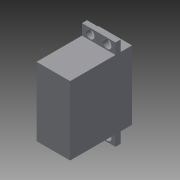
# Autodesk Inventor part: servo
Saved by Autodesk Inventor 2014 SP1 (Build 180222100, 222)
## iProperties
Created: 2014-03-28
Part Number: servo
Material: Générique
Document SubType Name: Modeling
Designer: astralien3000
Density: 1 g/cm^3
Appearance: Par défaut
length: 40,600 mm
width: 19,800 mm
axe_dist: 10,000 mm
d3: 9,900 mm
height: 36,600 mm
d5: 0,00 deg
handle_height: 26,800 mm
handle_thickness: 3,000 mm
handle_length: 6,400 mm
d9: 0,00 deg
d10: 26,800 mm
d11: 3,000 mm
d12: 6,400 mm
d13: 0,00 deg
d14: 9,900 mm
hole_dist: 5,000 mm
d16: 3,200 mm
hole_diameter: 5,000 mm
d19: 0,00 deg
d20: 9,900 mm
d21: 3,200 mm
d22: 5,000 mm
d23: 5,000 mm
d25: 0,00 deg
d26: 9,900 mm
d27: 5,000 mm
d28: 3,200 mm
d29: 5,000 mm
d31: 0,00 deg
d32: 9,900 mm
d33: 5,000 mm
d34: 5,000 mm
d35: 3,200 mm
d37: 0,00 deg
axe_diameter: 6,000 mm
axe_height: 6,700 mm
d40: 0,00 deg
d41: 10,000 mm
Author: astralien3000
Autodesk Inventor part; units mm, degrees
ref_plane "YZ Plane" through (0, 0, 0) normal (1, 0, 0) x (0, 1, 0)
ref_plane "XZ Plane" through (0, 0, 0) normal (0, 1, 0) x (-1, 0, 0)
ref_plane "XY Plane" through (0, 0, 0) normal (0, 0, 1) x (1, 0, 0)
sketch "servo_base" plane through (0, 0, 0) normal (0, 1, 0) x (-1, 0, 0)
  line L0 (-9.9, 10) -> (9.9, 10)
  line L1 (9.9, 10) -> (9.9, -30.6)
  line L2 (9.9, -30.6) -> (-9.9, -30.6)
  line L3 (-9.9, -30.6) -> (-9.9, 10)
  point P0 (0, 0)
  dimension "length" = 40.6
  dimension "width" = 19.8
  dimension "axe_dist" = 10
  dimension "d3" = 9.9
  constraints: 8 end point, 2 parallel, 1 horizontal, 1 perpendicular
  measures "length" distance of L0.end L1.end
  measures "width" distance of L0.start L0.end
  measures "axe_dist" distance from line of L0 point (0, 0)
  measures "d3" distance from line of L1 point (0, 0)
extrude "servo_body" add sketch "servo_base" along normal blind 36.6
sketch "handle1_base" plane through (-9.9, 0, 10) normal (0, 0, 1) x (1, 0, 0)
  line L0 (19.8, 0) -> (0, 0) projected
  line L1 (19.8, 0) -> (19.8, 36.6) projected
  line L2 (0, 0) -> (0, 36.6) projected
  line L3 (0, 26.8) -> (19.8, 26.8)
  line L4 (19.8, 26.8) -> (19.8, 29.8)
  line L5 (19.8, 29.8) -> (0, 29.8)
  line L6 (0, 29.8) -> (0, 26.8)
  point P0 (9.9, 0)
  dimension "handle_height" = 26.8
  dimension "handle_thickness" = 3
  constraints: 8 end point, 2 parallel, 2 point on line, 1 horizontal, 1 perpendicular
  measures "handle_height" distance between parallel lines of L0 L3
  measures "handle_thickness" distance between parallel lines of L3 L5
extrude "handle1" add sketch "handle1_base" along normal blind 6.4 contours L3 L2 L5 L1
sketch "handle2_base" plane through (9.9, 0, -30.6) normal (0, 0, -1) x (-1, 0, 0)
  line L0 (19.8, 0) -> (0, 0) projected
  line L1 (19.8, 0) -> (19.8, 36.6) projected
  line L2 (0, 0) -> (0, 36.6) projected
  line L3 (0, 26.8) -> (19.8, 26.8)
  line L4 (19.8, 26.8) -> (19.8, 29.8)
  line L5 (19.8, 29.8) -> (0, 29.8)
  line L6 (0, 29.8) -> (0, 26.8)
  point P0 (9.9, 0)
  dimension "d10" = 26.8
  dimension "d11" = 3
  constraints: 8 end point, 2 parallel, 2 point on line, 1 horizontal, 1 perpendicular
  measures "d10" distance between parallel lines of L0 L3
  measures "d11" distance between parallel lines of L3 L5
extrude "handle2" add sketch "handle2_base" along normal blind 6.4 contours L3 L2 L5 L1
sketch "hole1_right_base" plane through (-9.9, 29.8, 10) normal (0, 1, 0) x (1, 0, 0)
  line L0 (19.8, -6.4) -> (0, -6.4) projected
  line L1 (19.8, 0) -> (19.8, -6.4) projected
  line L2 (0, 0) -> (9.9, 0)
  line L3 (9.9, 0) -> (9.9, -6.4)
  line L4 (9.9, -6.4) -> (0, -6.4)
  line L5 (0, -6.4) -> (0, 0)
  circle A0 centre (4.9, -3.2) radius 2.5
  point P0 (9.9, 10)
  dimension "d14" = 9.9
  dimension "hole_dist" = 5
  dimension "d16" = 3.2
  dimension "hole_diameter" = 5
  constraints: 8 end point, 2 parallel, 1 centre point, 1 horizontal, 1 midpoint, 1 perpendicular
  measures "d14" distance between parallel lines of L1 L3
  measures "hole_dist" distance from line of L3 A0.centre
  measures "d16" distance from line of L0 A0.centre
  measures "hole_diameter" diameter of A0
extrude "hole1_rigth" cut sketch "hole1_right_base" against normal up to next contours A0
sketch "hole1_left_base" plane through (-9.9, 29.8, 10) normal (0, 1, 0) x (1, 0, 0)
  line L0 (0, 0) -> (0, -6.4) projected
  line L1 (19.8, -6.4) -> (0, -6.4) projected
  line L2 (19.8, 0) -> (9.9, 0)
  line L3 (9.9, 0) -> (9.9, -6.4)
  line L4 (9.9, -6.4) -> (19.8, -6.4)
  line L5 (19.8, -6.4) -> (19.8, 0)
  circle A0 centre (14.9, -3.2) radius 2.5
  point P0 (9.9, 10)
  dimension "d20" = 9.9
  dimension "d21" = 3.2
  dimension "d22" = 5
  dimension "d23" = 5
  constraints: 8 end point, 2 parallel, 1 centre point, 1 horizontal, 1 midpoint, 1 perpendicular
  measures "d20" distance between parallel lines of L0 L3
  measures "d21" distance from line of L1 A0.centre
  measures "d22" distance from line of L3 A0.centre
  measures "d23" diameter of A0
extrude "hole1_left" cut sketch "hole1_left_base" against normal up to next contours A0
sketch "hole2_right_base" plane through (-9.9, 29.8, -30.6) normal (0, 1, 0) x (1, 0, 0)
  line L0 (19.8, 0) -> (0, 0) projected
  line L1 (19.8, 0) -> (19.8, 6.4) projected
  line L2 (0, 6.4) -> (19.8, 6.4) projected
  line L3 (0, 6.4) -> (9.9, 6.4)
  line L4 (9.9, 6.4) -> (9.9, 0)
  line L5 (9.9, 0) -> (0, 0)
  line L6 (0, 0) -> (0, 6.4)
  circle A0 centre (4.9, 3.2) radius 2.5
  point P0 (9.9, -30.6)
  dimension "d26" = 9.9
  dimension "d27" = 5
  dimension "d28" = 3.2
  dimension "d29" = 5
  constraints: 8 end point, 2 parallel, 1 centre point, 1 horizontal, 1 midpoint, 1 perpendicular
  measures "d26" distance between parallel lines of L1 L4
  measures "d27" distance from line of L4 A0.centre
  measures "d28" distance from line of L2 A0.centre
  measures "d29" diameter of A0
extrude "hole2_right" cut sketch "hole2_right_base" against normal up to next contours A0
sketch "hole2_left_base" plane through (-9.9, 29.8, -30.6) normal (0, 1, 0) x (1, 0, 0)
  line L0 (19.8, 0) -> (0, 0) projected
  line L1 (0, 6.4) -> (19.8, 6.4) projected
  line L2 (0, 0) -> (0, 6.4) projected
  line L3 (19.8, 6.4) -> (9.9, 6.4)
  line L4 (9.9, 6.4) -> (9.9, 0)
  line L5 (9.9, 0) -> (19.8, 0)
  line L6 (19.8, 0) -> (19.8, 6.4)
  circle A0 centre (14.9, 3.2) radius 2.5
  point P0 (9.9, -30.6)
  dimension "d32" = 9.9
  dimension "d33" = 5
  dimension "d34" = 5
  dimension "d35" = 3.2
  constraints: 8 end point, 2 parallel, 1 centre point, 1 horizontal, 1 midpoint, 1 perpendicular
  measures "d32" distance between parallel lines of L2 L4
  measures "d33" diameter of A0
  measures "d34" distance from line of L4 A0.centre
  measures "d35" distance from line of L1 A0.centre
extrude "hole2_left" cut sketch "hole2_left_base" against normal up to next contours A0
sketch "axe_base" plane through (0, 36.6, 0) normal (0, 1, 0) x (1, 0, 0)
  circle A0 centre (0, 0) radius 3
  line L0 (-9.9, -10) -> (9.9, -10) projected
  line L1 (0, 0) -> (0, -10) construction
  dimension "axe_diameter" = 6
  dimension "d41" = 10
  constraints: 2 end point, 1 centre point, 1 coincident, 1 midpoint
  measures "axe_diameter" diameter of A0
  measures "d41" distance of L1.start L1.end
extrude "axe" add sketch "axe_base" along normal blind 6.7
equation "\"d3\" = 0.5 * width"
equation "\"d10\" = handle_height"
equation "\"d11\" = handle_thickness"
equation "\"d12\" = handle_length"
equation "\"d14\" = 0.5 * width"
equation "\"d16\" = 0.5 * handle_length"
equation "\"d18\" = handle_length"
equation "\"d20\" = 0.5 * width"
equation "\"d21\" = 0.5 * handle_length"
equation "\"d22\" = hole_dist"
equation "\"d23\" = hole_diameter"
equation "\"d24\" = handle_length"
equation "\"d26\" = 0.5 * width"
equation "\"d27\" = hole_dist"
equation "\"d28\" = 0.5 * handle_length"
equation "\"d29\" = hole_diameter"
equation "\"d30\" = handle_length"
equation "\"d32\" = 0.5 * width"
equation "\"d33\" = hole_diameter"
equation "\"d34\" = hole_dist"
equation "\"d35\" = 0.5 * handle_length"
equation "\"d36\" = handle_length"
equation "\"handle_length\" = 6.4"
